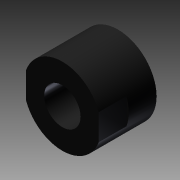
# Autodesk Inventor part: Suction Cup Part 3 1764
Saved by Autodesk Inventor 2011 (Build 150239000, 239)
## iProperties
Created: 2010-02-08
Part Number: Suction Cup Part 3 1764
Document SubType Name: Modeling
Designer: clee1
Density: 1 g/cm^3
Author: clee1
Autodesk Inventor part; units mm, degrees
ref_plane "YZ Plane" through (0, 0, 0) normal (1, 0, 0) x (0, 1, 0)
ref_plane "XZ Plane" through (0, 0, 0) normal (0, 1, 0) x (-1, 0, 0)
ref_plane "XY Plane" through (0, 0, 0) normal (0, 0, 1) x (1, 0, 0)
sketch "Sketch1" plane through (0, 0, 0) normal (0, 0, 1) x (1, 0, 0)
  circle A0 centre (0, 0) radius 11.4681
  circle A1 centre (0, 0) radius 5.3975
  dimension "d0" = 10.795
  dimension "d1" = 22.9362
  constraints: 2 centre point, 2 coincident
  measures "d0" diameter of A1
  measures "d1" diameter of A0
extrude "Extrusion1" add sketch "Sketch1" along normal blind 8.255
sketch "Sketch2" plane through (0, 0, 8.255) normal (0, 0, 1) x (1, 0, 0)
  circle A0 centre (0, 0) radius 5.3975 projected
  circle A1 centre (0, 0) radius 11.4681 projected
  circle A2 centre (0, 0) radius 11.4681
  line L0 (-10.795, 3.8711) -> (-10.795, -3.8711)
  line L1 (10.795, 3.8711) -> (10.795, -3.8711)
  dimension "d4" = 21.59
  constraints: 8 point on circle, 4 end point, 2 vertical, 1 centre point, 1 coincident, 1 concentric, 1 parallel
  measures "d4" distance between parallel lines of L1 L0
extrude "Extrusion2" add sketch "Sketch2" along normal blind 8.255 contours L1 A1 L0
body "Solid1"
